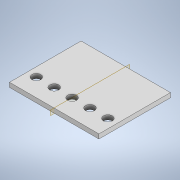
# Autodesk Inventor part: 5-holes
Saved by Autodesk Inventor 2020.2 (Build 242310000, 310)
## iProperties
Created: 2020-03-13
Part Number: 5-holes
Material: Generic
Document SubType Name: Modeling
Designer: robst
Density: 1 g/cm^3
Appearance: Default
Author: robst
Autodesk Inventor part; units mm, degrees
ref_plane "XZ Plane" through (0, 0, 0) normal (0, 1, 0) x (-1, 0, 0)
ref_plane "XY Plane" through (0, 0, 0) normal (0, 0, 1) x (1, 0, 0)
sketch "Sketch1" plane through (0, 0, 0) normal (0, 1, 0) x (-1, 0, 0)
  line L0 (63.5, 50.8) -> (-63.5, 50.8)
  line L1 (-63.5, 50.8) -> (-63.5, -50.8)
  line L2 (-63.5, -50.8) -> (63.5, -50.8)
  line L3 (63.5, -50.8) -> (63.5, 50.8)
  line L4 (63.5, 50.8) -> (-63.5, -50.8) construction
  line L5 (-63.5, 50.8) -> (63.5, -50.8) construction
  point P0 (0, 0)
  dimension "d3" = 101.6
  dimension "d13" = 127
  constraints: 12 end point, 2 midpoint, 2 parallel, 1 horizontal, 1 perpendicular
  measures "d3" distance of L2.end L0.start
  measures "d13" distance of L1.end L2.end
extrude "Extrusion1" add sketch "Sketch1" against normal blind 6.35
sketch "Sketch3" plane through (0, 0, 0) normal (0, 1, 0) x (1, 0, 0)
  line L0 (-63.5, -50.8) -> (-63.5, 50.8) construction
  line L1 (-63.5, -25.4) -> (63.5, -25.4) construction
  line L2 (63.5, 50.8) -> (63.5, -50.8) construction
  line L3 (63.5, 50.8) -> (-63.5, 50.8) construction
  circle A0 centre (-50.8, -25.4) radius 6.35
  circle A1 centre (-25.4, -25.4) radius 6.35
  circle A2 centre (0, -25.4) radius 6.35
  circle A3 centre (25.4, -25.4) radius 6.35
  circle A4 centre (50.8, -25.4) radius 6.35
  point P0 (0, 0)
  dimension "d2" = 76.2
  dimension "d4" = 12.7
  dimension "d5" = 12.7
  dimension "d8" = 25.4
  constraints: 5 centre point, 3 point on line, 2 end point, 2 horizontal, 8 other
  measures "d2" distance between parallel lines of L1 L3
  measures "d4" diameter of A0
  measures "d5" distance from line of A0.centre L0
  measures "d8" distance of A0.centre A1.centre
extrude "Extrusion2" cut sketch "Sketch3" against normal through all
body "Solid1"
